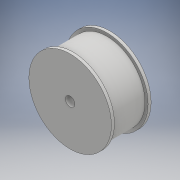
# Autodesk Inventor part: Kolo
Saved by Autodesk Inventor 2018 (Build 220112000, 112)
## iProperties
Created: 2019-08-04
Part Number: Kolo
Material: Ogólny
Document SubType Name: Modeling
Designer: Raven
Density: 1 g/cm^3
Appearance: Domyślna
Author: Raven
Autodesk Inventor part; units mm, degrees
ref_plane "YZ Plane" through (0, 0, 0) normal (1, 0, 0) x (0, 1, 0)
ref_plane "XZ Plane" through (0, 0, 0) normal (0, 1, 0) x (-1, 0, 0)
ref_plane "XY Plane" through (0, 0, 0) normal (0, 0, 1) x (1, 0, 0)
sketch "Szkic1" plane through (0, 0, 0) normal (0, 0, 1) x (1, 0, 0)
  line L0 (0, 0) -> (13.5, 0)
  line L1 (13.5, 0) -> (13.5, 1)
  line L2 (13.5, 1) -> (12.5, 1)
  line L3 (12.5, 1) -> (12.5, 12)
  line L4 (12.5, 12) -> (13.5, 12)
  line L5 (13.5, 12) -> (13.5, 13)
  line L6 (13.5, 13) -> (5.5, 13)
  line L7 (5.5, 13) -> (5.5, 7)
  line L8 (5.5, 7) -> (3.1, 7)
  line L9 (3.1, 7) -> (0, 7)
  line L10 (0, 7) -> (0, 0)
  dimension "d0" = 13.5
  dimension "d1" = 1
  dimension "d2" = 1
  dimension "d3" = 11
  dimension "d4" = 1
  dimension "d5" = 1
  dimension "d6" = 8
  dimension "d7" = 6
  dimension "d8" = 2.4
  constraints: 22 end point, 7 perpendicular, 2 horizontal, 2 point on line
  measures "d0" distance of L0.start L0.end
  measures "d1" distance of L0.end L1.end
  measures "d2" distance of L1.end L2.end
  measures "d3" distance of L2.end L3.end
  measures "d4" distance of L3.end L4.end
  measures "d5" distance of L4.end L5.end
  measures "d6" distance of L5.end L6.end
  measures "d7" distance of L6.end L7.end
  measures "d8" distance of L7.end L8.end
revolve "Obrót1" add sketch "Szkic1" angle 360 about axis through (0, 7, 0) along (0, -1, 0)
sketch "Szkic2" plane through (0, 7, 0) normal (0, 1, 0) x (1, 0, 0)
  circle A0 centre (0, 0) radius 5.5 projected
  circle A1 centre (0, 0) radius 1.55
  dimension "d10" = 3.1
  constraints: 1 centre point, 1 coincident
  measures "d10" diameter of A1
extrude "Wyciągnięcie proste1" cut sketch "Szkic2" against normal blind 10 contours A1
